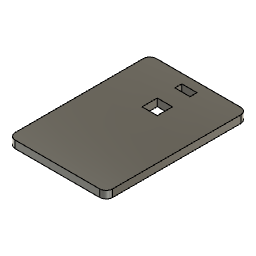
sughrue_b_card_to_cut (Autodesk Fusion 360 design; units mm, degrees)
Autodesk Fusion 360 part; units mm, degrees
sketch "Sketch1" plane through (0, 0, 0) normal (0, 0, 1) x (1, 0, 0)
  line L0 (4, 0) -> (56.35, 0)
  line L1 (60.35, 4) -> (60.35, 83.39)
  line L2 (56.35, 87.39) -> (4, 87.39)
  line L3 (0, 83.39) -> (0, 4)
  arc A0 (4, 87.39) -> (0, 83.39) centre (4, 83.39) ccw
  arc A1 (60.35, 83.39) -> (56.35, 87.39) centre (56.35, 83.39) ccw
  arc A2 (56.35, 0) -> (60.35, 4) centre (56.35, 4) ccw
  arc A3 (0, 4) -> (4, 0) centre (4, 4) ccw
  line L4 (30.175, 81.69) -> (25.475, 81.69)
  line L5 (30.175, 81.69) -> (34.875, 81.69)
  line L6 (30.175, 77.39) -> (25.475, 77.39)
  line L7 (30.175, 77.39) -> (34.875, 77.39)
  line L8 (25.475, 81.69) -> (25.475, 77.39)
  line L9 (34.875, 81.69) -> (34.875, 77.39)
  line L10 (34.875, 66.4941) -> (25.475, 66.4941)
  line L11 (34.875, 57.0941) -> (25.475, 57.0941)
  line L12 (34.875, 57.0941) -> (34.875, 61.7941)
  line L13 (34.875, 61.7941) -> (34.875, 66.4941)
  line L14 (25.475, 57.0941) -> (25.475, 61.7941)
  line L15 (25.475, 61.7941) -> (25.475, 66.4941)
  point P0 (60.35, 0)
  point P1 (0, 87.39)
  dimension "d6" = 60.35
  dimension "d7" = 87.39
  dimension "d9" = 4
  dimension "d10" = 4
  dimension "d11" = 4
  dimension "d12" = 4
  dimension "d16" = 4.3
  constraint horizontal L0
  constraint vertical L1
  constraint horizontal L2
  constraint vertical L3
  constraint coincident P1 L2
  constraint coincident P1 L3
  constraint tangent L2 A0
  constraint tangent L3 A0
  constraint tangent L1 A1
  constraint tangent L2 A1
  constraint coincident P0 L0
  constraint coincident P0 L1
  constraint tangent L0 A2
  constraint tangent L1 A2
  constraint coincident origin L0
  constraint coincident origin L3
  constraint tangent L0 A3
  constraint tangent L3 A3
  constraint perpendicular L3 L4
  constraint perpendicular L1 L5
  constraint coincident L12 L11.start
  measures "d6" distance of origin P0
  measures "d7" distance of origin P1
  measures "d9" radius of A0
  measures "d10" radius of A1
  measures "d11" radius of A2
  measures "d12" radius of A3
  measures "d16" distance of L6.start L4.start
extrude "Extrude2" add sketch "Sketch1" along normal blind 4.6
extrude "Extrude1" [suppressed]
equation "long_side_length = 87.39 mm"
equation "short_side_length = 60.35 mm"
equation "kerf = 0.6 mm"
equation "notch_depth = 10 mm"
equation "thickness = 4.6 mm"
equation "d6 = short_side_length"
equation "d7 = long_side_length"
equation "rounded_edge_length = 4 mm"
equation "d9 = rounded_edge_length"
equation "d10 = rounded_edge_length"
equation "d11 = rounded_edge_length"
equation "d12 = rounded_edge_length"
equation "d16 = thickness - ( kerf / 2 )"
equation "d22 = thickness"
equation "d43 = thickness"
